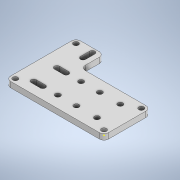
# Autodesk Inventor part: X_Carriage_Plate
Saved by Autodesk Inventor 2021 (Build 250183000, 183)
## iProperties
Created: 2021-06-13
Part Number: X_Carriage_Plate
Material: Generic
Document SubType Name: Modeling
Designer: Jorian Brusind
Density: 1 g/cm^3
Appearance: Default
Author: Jorian Brusind
Autodesk Inventor part; units mm, degrees
ref_plane "YZ Plane" through (0, 0, 0) normal (1, 0, 0) x (0, 1, 0)
ref_plane "XZ Plane" through (0, 0, 0) normal (0, 1, 0) x (-1, 0, 0)
ref_plane "XY Plane" through (0, 0, 0) normal (0, 0, 1) x (1, 0, 0)
sketch "Sketch1" plane through (0, 0, 0) normal (0, 1, 0) x (-1, 0, 0)
  line L0 (0, 0) -> (105, 0)
  line L1 (105, 0) -> (105, -50)
  line L2 (105, -50) -> (0, -50)
  line L3 (0, -50) -> (0, 0)
  line L4 (0, 0) -> (0, -16.6667)
  line L5 (0, -16.6667) -> (11, -16.6667)
  dimension "d0" = 105
  dimension "d1" = 50
  dimension "d2" = 16.6667
  dimension "d3" = 11
  constraints: 12 end point, 2 parallel, 2 perpendicular, 1 horizontal, 1 point on line
  measures "d0" distance of L1.end L2.end
  measures "d1" distance of L0.end L1.end
  measures "d2" distance of L0.start L4.end
  measures "d3" distance of L4.end L5.end
extrude "Extrusion1" add sketch "Sketch1" along normal blind 6
sketch "Sketch3" plane through (0, 6, 0) normal (0, 1, 0) x (1, 0, 0)
  circle A0 centre (-20, 12.5) radius 2.75
  line L0 (0, 0) -> (0, 50) projected
  line L1 (-105, 0) -> (0, 0) projected
  circle A1 centre (-20, 37.5) radius 2.75
  dimension "d21" = 5.5
  dimension "d22" = 20
  dimension "d23" = 12.5
  dimension "d26" = 25
  constraints: 2 centre point, 1 vertical, 2 other
  measures "d21" diameter of A0
  measures "d22" distance from line of L0 A0.centre
  measures "d23" distance from line of L1 A0.centre
  measures "d26" distance of A0.centre A1.centre
extrude "Extrusion3" cut sketch "Sketch3" against normal through all
sketch "Sketch4" plane through (0, 6, 0) normal (0, 1, 0) x (1, 0, 0)
  circle A0 centre (-20, 12.5) radius 2.75 projected
  line L0 (-20, 12.5) -> (-78, 12.5)
  line L1 (-78, 12.5) -> (-88, 12.5) construction
  line L2 (-78, 15.25) -> (-88, 15.25)
  line L3 (-88, 9.75) -> (-78, 9.75)
  arc A1 (-78, 9.75) -> (-78, 15.25) centre (-78, 12.5) ccw
  arc A2 (-88, 15.25) -> (-88, 9.75) centre (-88, 12.5) ccw
  point P0 (0, 0)
  point P1 (-83, 12.5)
  dimension "d33" = 58
  dimension "d34" = 10
  dimension "d35" = 5.5
  constraints: 10 end point, 4 point on circle, 4 tangent, 2 centre point, 2 horizontal, 1 midpoint, 1 parallel
  measures "d33" distance of L0.start L0.end
  measures "d34" distance of L0.end L1.end
  measures "d35" diameter of A2
extrude "Extrusion4" cut sketch "Sketch4" against normal through all contours A1 L3 A2 L2
pattern_linear "Rectangular Pattern2" count 2 spacing 25 along (0, 0, -1) of "Extrusion4"
sketch "Sketch5" plane through (0, 0, -50) normal (0, 0, -1) x (-1, 0, 0)
  line L0 (105, 0) -> (105, 6) projected
  line L1 (105, 0) -> (0, 0) projected
  line L2 (105, 6) -> (75, 6)
  line L3 (75, 6) -> (75, 0)
  line L4 (75, 0) -> (105, 0)
  line L5 (105, 0) -> (105, 6)
  dimension "d45" = 30
  constraints: 8 end point, 2 parallel, 1 horizontal, 1 perpendicular, 1 point on line
  measures "d45" distance of L4.end L3.end
extrude "Extrusion5" add sketch "Sketch5" along normal blind 25
sketch "Sketch6" plane through (0, 6, 0) normal (0, 1, 0) x (1, 0, 0)
  line L0 (-83, 60.5) -> (-83, 70.5) construction
  line L1 (-80.25, 60.5) -> (-80.25, 70.5)
  line L2 (-85.75, 70.5) -> (-85.75, 60.5)
  arc A0 (-85.75, 60.5) -> (-80.25, 60.5) centre (-83, 60.5) ccw
  arc A1 (-80.25, 70.5) -> (-85.75, 70.5) centre (-83, 70.5) ccw
  line L3 (-75, 50) -> (-75, 75) projected
  arc A2 (-88, 40.25) -> (-88, 34.75) centre (-88, 37.5) ccw projected
  point P0 (0, 0)
  point P1 (-83, 65.5)
  dimension "d48" = 10
  dimension "d49" = 5.5
  dimension "d50" = 8
  dimension "d51" = 28
  constraints: 8 end point, 4 point on circle, 4 tangent, 2 centre point, 1 midpoint, 1 parallel, 1 vertical
  measures "d48" distance of L0.start L0.end
  measures "d49" diameter of A1
  measures "d50" distance from line of L3 point (-83, 65.5)
  measures "d51" vertical distance of A2.centre point (-83, 65.5)
extrude "Extrusion6" cut sketch "Sketch6" against normal through all
fillet "Fillet2" radius 5 6 edges at (-105, 3, 0) (0, 3, 0) (-75, 3, -75) (-105, 3, -75) (0, 3, -50) (-75, 3, -50)
sketch "Sketch7" plane through (0, 6, 0) normal (0, 1, 0) x (1, 0, 0)
  circle A0 centre (-20, 12.5) radius 2.75 projected
  line L0 (-20, 12.5) -> (-42, 12.5)
  line L1 (-42, 12.5) -> (-62, 12.5)
  circle A1 centre (-62, 12.5) radius 2.75
  circle A2 centre (-42, 12.5) radius 2.75
  line L2 (0, 5) -> (0, 45) projected
  line L3 (0, 0) -> (0, 45)
  circle A3 centre (-42, 37.5) radius 2.75
  circle A4 centre (-62, 37.5) radius 2.75
  dimension "d55" = 22
  dimension "d56" = 20
  dimension "d57" = 5.5
  dimension "d58" = 5.5
  dimension "d61" = 25
  constraints: 6 end point, 4 centre point, 2 coincident, 2 horizontal, 1 collinear, 1 vertical, 4 other
  measures "d55" distance of L0.start L0.end
  measures "d56" distance of L0.end L1.end
  measures "d57" diameter of A1
  measures "d58" diameter of A2
  measures "d61" distance of A2.centre A3.centre
extrude "Extrusion7" cut sketch "Sketch7" against normal through all contours A1 | A2 L1 L0 | L0 L1 A2 | A3 | A4
sketch "Sketch9" plane through (0, 6, 0) normal (0, 1, 0) x (1, 0, 0)
  point P0 (0, 0)
sketch "Sketch10" plane through (0, 6, 0) normal (0, 1, 0) x (1, 0, 0)
  circle A0 centre (-100, 70) radius 2.75
  line L0 (-100, 75) -> (-80, 75) projected
  line L1 (-105, 5) -> (-105, 70) projected
  circle A1 centre (-100, 5) radius 2.75
  line L2 (-100, 0) -> (-5, 0) projected
  circle A2 centre (-5, 45) radius 2.75
  line L3 (-5, 50) -> (-70, 50) projected
  line L4 (0, 5) -> (0, 45) projected
  circle A3 centre (-5, 5) radius 2.75
  point P0 (0, 0)
  dimension "d70" = 5.5
  dimension "d71" = 5
  dimension "d72" = 5
  dimension "d73" = 5.5
  dimension "d74" = 5
  dimension "d75" = 5
  dimension "d76" = 5.5
  dimension "d77" = 5
  dimension "d78" = 5
  dimension "d79" = 5.5
  dimension "d80" = 5
  dimension "d81" = 5
  constraints: 4 centre point
  measures "d70" diameter of A0
  measures "d71" distance from line of L0 A0.centre
  measures "d72" distance from line of L1 A0.centre
  measures "d73" diameter of A1
  measures "d74" distance from line of L2 A1.centre
  measures "d75" distance from line of L1 A1.centre
  measures "d76" diameter of A2
  measures "d77" distance from line of L3 A2.centre
  measures "d78" distance from line of L4 A2.centre
  measures "d79" diameter of A3
  measures "d80" distance from line of L4 A3.centre
  measures "d81" distance from line of L2 A3.centre
extrude "Extrusion9" cut sketch "Sketch10" against normal through all
body "Solid1"
